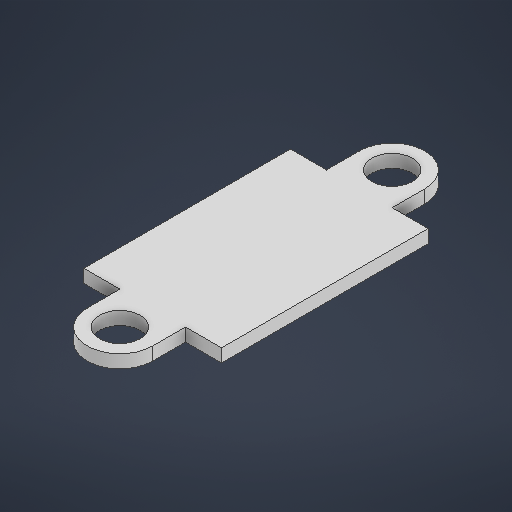
# Autodesk Inventor part: 1XV2
Saved by Autodesk Inventor 2026.2 (Build 302298010, 298A)
## iProperties
Created: 2026-06-28
Part Number: 1XV2
Material: Ogólny
Document SubType Name: Modeling
Designer: karol
Density: 1 g/cm^3
Appearance: Domyślna
Author: karol
Autodesk Inventor part; units mm, degrees
ref_plane "YZ Plane" through (0, 0, 0) normal (1, 0, 0) x (0, 1, 0)
ref_plane "XZ Plane" through (0, 0, 0) normal (0, 1, 0) x (-1, 0, 0)
ref_plane "XY Plane" through (0, 0, 0) normal (0, 0, 1) x (1, 0, 0)
sketch "Szkic1" plane through (0, 0, 0) normal (0, 1, 0) x (-1, 0, 0)
  line L0 (0, 0) -> (10.5, 0)
  line L1 (10.5, 0) -> (10.5, -15.75)
  line L2 (10.5, -15.75) -> (0, -15.75)
  line L3 (0, -15.75) -> (0, 0)
  line L4 (7.75, -15.75) -> (2.75, -15.75)
  line L5 (2.75, -15.75) -> (2.75, -20.75)
  line L6 (2.75, -20.75) -> (7.75, -20.75)
  line L7 (7.75, -20.75) -> (7.75, -15.75)
  line L8 (7.75, 0) -> (2.75, 0)
  line L9 (2.75, 0) -> (2.75, 5)
  line L10 (2.75, 5) -> (7.75, 5)
  line L11 (7.75, 5) -> (7.75, 0)
  circle A0 centre (5.25, 2.5) radius 1.55
  circle A1 centre (5.25, -18.25) radius 1.55
  point P0 (5.25, -20.75)
  point P1 (7.75, -18.25)
  point P2 (5.25, 5)
  point P3 (7.75, 2.5)
  dimension "d0" = 10.5
  dimension "d1" = 15.75
  dimension "d2" = 5
  dimension "d3" = 5
  dimension "d4" = 2.75
  dimension "d5" = 5
  dimension "d6" = 5
  dimension "d7" = 2.75
  dimension "d8" = 3.1
  dimension "d9" = 3.1
  dimension "d10" = 2.5
  dimension "d11" = 2.5
  dimension "d12" = 2.5
  dimension "d13" = 2.5
  constraints: 24 end point, 6 parallel, 4 midpoint, 3 horizontal, 3 perpendicular, 2 centre point, 2 point on line
  measures "d0" distance of L1.end L2.end
  measures "d1" distance of L0.end L1.end
  measures "d2" distance of L6.end L5.end
  measures "d3" distance of L5.end L4.end
  measures "d4" distance between parallel lines of L1 L7
  measures "d5" distance of L9.end L10.end
  measures "d6" distance of L8.end L9.end
  measures "d7" distance between parallel lines of L1 L11
  measures "d8" diameter of A0
  measures "d9" diameter of A1
  measures "d10" distance of point (5.25, -20.75) A1.centre
  measures "d11" distance of point (7.75, -18.25) A1.centre
  measures "d12" distance of point (5.25, 5) A0.centre
  measures "d13" distance of point (7.75, 2.5) A0.centre
extrude "Wyciągnięcie proste1" add sketch "Szkic1" along normal blind 1
fillet "Zaokrąglenie1" radius 2.5 4 edges at (-2.75, 0.5, 5) (-7.75, 0.5, 5) (-2.75, 0.5, -20.75) (-7.75, 0.5, -20.75)
